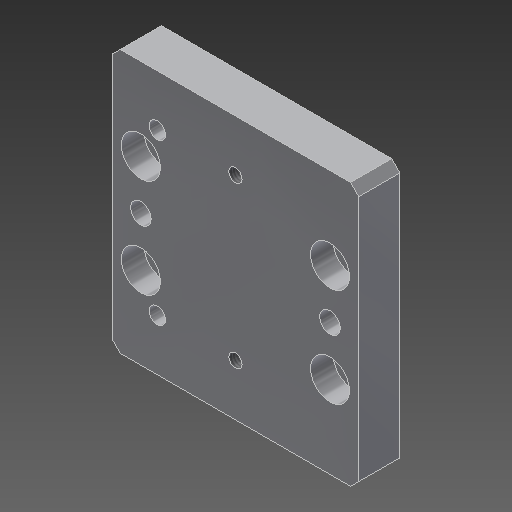
# Autodesk Inventor part: 03
Saved by Autodesk Inventor 2021.1 (Build 251245010, 245A)
## iProperties
Created: 2008-11-14
Part Number: 03
Document SubType Name: Modeling
Density: 2.71 g/cm^3
Material: A5052
Mass: 104.064 g
Surface Area: 101.6 cm^2
Volume: 38.4 cm^3
Appearance: アルミニウム - フラット
個数: 1
尺度: 1:1
Title: プレート
Autodesk Inventor part; units mm, degrees
ref_plane "YZ Plane" through (0, 0, 0) normal (1, 0, 0) x (0, 1, 0)
ref_plane "XZ Plane" through (0, 0, 0) normal (0, 1, 0) x (-1, 0, 0)
ref_plane "XY Plane" through (0, 0, 0) normal (0, 0, 1) x (1, 0, 0)
sketch "スケッチ1" plane through (0, 0, 0) normal (0, 0, 1) x (1, 0, 0)
  line L0 (-30, -32) -> (30, -32)
  line L1 (30, -32) -> (30, 32)
  line L2 (30, 32) -> (-30, 32)
  line L3 (-30, 32) -> (-30, -32)
  point P0 (0, 0)
  point P1 (0, -32)
  point P2 (-30, 0)
  dimension "d0" = 60
  dimension "d1" = 64
  constraints: 8 end point, 2 midpoint, 2 parallel, 1 horizontal, 1 horizontal alignment, 1 perpendicular, 1 vertical alignment
  measures "d0" distance of L0.start L0.end
  measures "d1" distance of L2.end L0.start
extrude "押し出し1" add sketch "スケッチ1" along normal blind 10
sketch "スケッチ2" plane through (0, 0, 10) normal (0, 0, 1) x (1, 0, 0)
  point P0 (0, 0)
  point P1 (-23, -12)
  dimension "d4" = 23
  dimension "d5" = 12
  measures "d4" horizontal distance of point (-23, -12) point (0, 0)
  measures "d5" vertical distance of point (-23, -12) point (0, 0)
hole "穴1" at (-23, -12, 10) direction (0, 0, -1) diameter 5.5 end through all counterbore diameter 9.5 counterbore depth 5.5
pattern_linear "矩形状パターン1" count 2 spacing 24 along (0, 1, 0) count 2 spacing 46 along (1, 0, 0) of "穴1"
sketch "スケッチ3" plane through (0, 0, 10) normal (0, 0, 1) x (1, 0, 0)
  circle A0 centre (23, -12) radius 4.75 projected
  circle A1 centre (-23, -12) radius 4.75 projected
  point P0 (0, 0)
  point P1 (-23, 0)
  point P2 (23, 0)
  constraints: 2 horizontal alignment, 2 vertical alignment
hole "穴2" at (-23, 0, 10) at (23, 0, 10) direction (0, 0, -1) diameter 5 end through all
sketch "スケッチ4" plane through (0, 0, 10) normal (0, 0, 1) x (1, 0, 0)
  point P0 (0, 0)
  point P1 (0, 19.5)
  point P2 (0, -19.5)
  dimension "d26" = 19.5
  dimension "d27" = 19.5
  constraints: 2 vertical alignment
  measures "d26" distance of point (0, -19.5) point (0, 0)
  measures "d27" distance of point (0, 19.5) point (0, 0)
hole "穴3" at (0, 19.5, 10) at (0, -19.5, 10) direction (0, 0, -1) diameter 3.242 end through all thread size "M4x0.7" class "6H" standard "ANSI Metric M Profile"
sketch "スケッチ5" plane through (0, 0, 10) normal (0, 0, 1) x (1, 0, 0)
  circle A0 centre (0, -19.5) radius 1.621 projected
  circle A1 centre (0, 19.5) radius 1.621 projected
  point P0 (0, 0)
  point P1 (-19, 19.5)
  point P2 (-19, -19.5)
  dimension "d35" = 19
  constraints: 2 horizontal alignment, 1 vertical alignment
  measures "d35" distance of point (-19, -19.5) A0.centre
hole "穴4" at (-19, 19.5, 10) at (-19, -19.5, 10) direction (0, 0, -1) diameter 4 end through all
chamfer "面取り1" distance 2 angle 45 4 edges at (30, 32, 5) (30, -32, 5) (-30, -32, 5) (-30, 32, 5)
equation "\"d27\" = d26"
